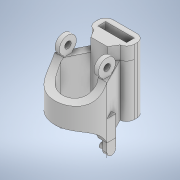
# Autodesk Inventor part: 손가락_중간
Saved by Autodesk Inventor 2022 (Build 260153000, 153)
## iProperties
Created: 2023-11-18
Part Number: 손가락_중간
Material: 일반
Document SubType Name: Modeling
Designer: USER
Density: 1 g/cm^3
Appearance: 기본값
Author: USER
Autodesk Inventor part; units mm, degrees
ref_plane "YZ Plane" through (0, 0, 0) normal (1, 0, 0) x (0, 1, 0)
ref_plane "XZ Plane" through (0, 0, 0) normal (0, 1, 0) x (-1, 0, 0)
sketch "스케치1" plane through (0, 0, 0) normal (0, 1, 0) x (-1, 0, 0)
  line L0 (0, 0) -> (0, -20)
  line L1 (0, -10) -> (-10, -10)
  line L2 (0, -20) -> (-5, -20)
  line L3 (-5, -20) -> (-10, -10)
  arc A0 (0, 0) -> (-10, -10) centre (0, -10) ccw
  line L4 (0, -20) -> (5, -20)
  line L5 (5, -20) -> (10, -10)
  arc A1 (10, -10) -> (0, 0) centre (0, -10) ccw
  dimension "d0" = 20
  dimension "d1" = 10
  dimension "d2" = 5
  constraints: 12 end point, 4 point on circle, 2 centre point, 2 horizontal, 2 symmetric about line, 1 coincident, 1 midpoint, 1 point on line, 1 vertical, 1 other
  measures "d0" distance of L0.start L0.end
  measures "d1" distance of L1.end L1.start
  measures "d2" distance of L0.end L2.end
extrude "돌출1" add sketch "스케치1" along normal blind 20
sketch "스케치2" plane through (0, 0, 0) normal (1, 0, 0) x (0, 1, 0)
  line L0 (0, 0) -> (20, 0) projected
  line L1 (20.0022, 0) -> (14.0022, 0)
  line L2 (25.6628, 0) -> (14.0022, 0)
  line L3 (10.0065, 0) -> (10.0065, 12.925)
  spline S0 degree 2 poles (14.0022, 0) (13.9613, -9.8069) (25.6628, -11.6913) knots 0 0 0 1 1 1
  line L4 (25.6628, -11.6913) -> (25.6628, 0)
  line L5 (0, -10) -> (20, -10) projected
  line L6 (0, -10) -> (28.6414, -10)
  line L7 (0, -10) -> (-10.0964, -10)
  line L8 (-5.6498, 0) -> (6.0108, 0)
  spline S1 degree 2 poles (6.0108, 0) (6.0517, -9.8069) (-5.6498, -11.6913) knots 0 0 0 1 1 1
  line L9 (-5.6498, -11.6913) -> (-5.6498, 0)
  point P0 (16.5578, -7.4686)
  point P1 (3.4551, -7.4686)
  point P2 (6.0108, 0)
  dimension "d5" = 6
  constraints: 16 end point, 4 symmetric about line, 3 point on line, 2 horizontal, 1 perpendicular, 1 vertical, 7 other
  measures "d5" distance of L1.start L1.end
shell "쉘1" thickness 3 removed faces 2 at (1.8644, 20, -8.0053) at (1.8644, 0, -8.0053)
extrude "돌출3" cut sketch "스케치2" along normal mid plane 30 contours L0 L1 L2 L4 L6 S0 | L6 L4 S0
sketch "스케치8" plane through (0, 20, 0) normal (0, 1, 0) x (1, 0, 0)
  arc A0 (-10, 10) -> (10, 10) centre (0, 10) ccw projected
  line L0 (-6.6459, 10) -> (-3.1459, 17) projected
  line L1 (-10, 10) -> (-6.6459, 10)
  line L2 (-8.3229, 10) -> (-8.3229, 13.3541)
  line L3 (-5, 20) -> (-10, 10) projected
  line L4 (-8.3229, 13.3541) -> (-6.6459, 13.3541)
  line L5 (-6.6459, 13.3541) -> (-6.6459, 10)
  line L6 (5, 20) -> (-5, 20) projected
  line L7 (0, 20) -> (0, 17)
  line L8 (-3.1459, 17) -> (3.1459, 17) projected
  line L9 (-8.3229, 10) -> (-6.6459, 10)
  line L10 (10, 10) -> (6.6459, 10)
  line L11 (8.3229, 10) -> (8.3229, 13.3541)
  line L12 (8.3229, 13.3541) -> (6.6459, 13.3541)
  line L13 (6.6459, 13.3541) -> (6.6459, 10)
  point P0 (0, 0)
  constraints: 20 end point, 4 symmetric about line, 3 horizontal, 3 midpoint, 1 perpendicular, 1 point on line, 1 vertical
extrude "돌출7" cut sketch "스케치2" along normal mid plane 30 contours L0 S1 L5 L7 L9 L8 | S1 L9 L7 L5
sketch "스케치9" plane through (0, 0, 0) normal (0, -1, 0) x (1, 0, 0)
  line L0 (9.9968, -10.0064) -> (5, -20) projected
  line L1 (6.6427, -10.0064) -> (3.1459, -17) projected
  line L2 (9.9968, -10.0064) -> (6.6427, -10.0064)
  line L3 (8.3198, -10.0064) -> (8.3198, -13.3605)
  line L4 (5, -20) -> (-5, -20) projected
  line L5 (0, -20) -> (0, -17)
  line L6 (-3.1459, -17) -> (3.1459, -17) projected
  line L7 (10, -10) -> (5, -20) projected
  line L8 (10, -10) -> (10, -13.3605)
  line L9 (10, -13.3605) -> (8.3198, -13.3605)
  line L10 (-9.9968, -10.0064) -> (-6.6427, -10.0064)
  line L11 (-5, -20) -> (-9.9968, -10.0064) projected
  line L12 (-9.9968, -10.0064) -> (-9.9968, -13.3605)
  line L13 (-9.9968, -13.3605) -> (-8.3198, -13.3605)
  line L14 (-8.3198, -13.3605) -> (-8.3198, -10.0064)
  point P0 (0, 0)
  constraints: 18 end point, 4 midpoint, 3 perpendicular, 3 symmetric about line, 2 vertical, 1 horizontal, 1 point on line
extrude "돌출8" add sketch "스케치8" along normal blind 5 contours L1 L2 L4 L5 | L10 L13 L12 L11
extrude "돌출9" add sketch "스케치9" along normal blind 5 contours L7 L8 L9 L0 | L0 L3 L2 | L10 L14 L11 | L11 L13 L12
sketch "스케치10" plane through (8.3229, 20, -10) normal (1, 0, 0) x (0, 0, -1)
  line L0 (10, 0) -> (3.3541, 0) projected
  line L1 (0, 5) -> (3.3541, 5)
  line L2 (3.3541, 5) -> (3.3541, 0)
  line L3 (3.3541, 0) -> (0, 0)
  line L4 (0, 0) -> (0, 5)
  circle A0 centre (1.6771, 3.3229) radius 3.25
  line L5 (3.3541, 0) -> (3.3541, 5) projected
  circle A1 centre (1.6771, 3.3229) radius 1.25
  point P0 (-10, -20)
  point P1 (0, 0.5391)
  point P2 (1.6771, 5)
  point P3 (3.3541, 0.5391)
  dimension "d28" = 6.5
  dimension "d29" = 2.5
  constraints: 8 end point, 2 centre point, 2 parallel, 1 coincident, 1 horizontal, 1 perpendicular
  measures "d28" diameter of A0
  measures "d29" diameter of A1
sketch "스케치11" plane through (0, 0, 0) normal (0, 1, 0) x (1, 0, 0)
  line L0 (-9.9968, 13.3605) -> (-8.3198, 13.3605) projected
  line L1 (-9.9968, 13.3605) -> (-8.3198, 13.3605)
  line L2 (-8.3198, 13.3605) -> (-9.9968, 10.0064) projected
  line L3 (-8.3198, 13.3605) -> (-9.9968, 10.0064)
  line L4 (-9.9968, 10.0064) -> (-9.9968, 13.3605) projected
  line L5 (-9.9968, 10.0064) -> (-9.9968, 13.3605)
  line L6 (8.3198, 13.3605) -> (10, 13.3605) projected
  line L7 (8.3198, 13.3605) -> (10, 13.3605)
  line L8 (9.9968, 10.0064) -> (8.3198, 13.3605) projected
  line L9 (10, 13.3605) -> (9.9968, 10.0064)
  line L10 (9.9968, 10.0064) -> (8.3198, 13.3605)
  point P0 (0, 0)
  constraints: 12 end point, 5 collinear
extrude "돌출10" add sketch "스케치11" along normal blind 8
sketch "스케치12" plane through (8.3198, 0, -13.3605) normal (-1, 0, 0) x (0, 0, 1)
  line L0 (0, 0) -> (3.3541, 0) projected
  line L1 (0, 0) -> (0, -5) projected
  line L2 (3.3541, 0) -> (0, 0)
  line L3 (0, 0) -> (0, -5)
  line L4 (0, -5) -> (3.3541, -5)
  line L5 (3.3541, -5) -> (3.3541, 0)
  circle A0 centre (1.6771, -3.3229) radius 1.6771
  line L6 (3.3541, 0) -> (3.3541, -5) projected
  line L7 (3.3541, -5) -> (0, -5) projected
  circle A1 centre (1.6771, -3.3229) radius 1
  point P0 (13.3605, 0)
  point P1 (3.3541, -3.3229)
  point P2 (1.6771, -5)
  point P3 (0, -3.3229)
  dimension "d32" = 2
  constraints: 8 end point, 2 centre point, 2 parallel, 2 tangent, 1 coincident, 1 horizontal, 1 perpendicular
  measures "d32" diameter of A1
extrude "돌출11" cut sketch "스케치12" along normal mid plane 100 contours A0 L4 L1 | L5 L4 A0
extrude "돌출12" add sketch "스케치12" along normal blind 2 contours A1
sketch "스케치13" plane through (-8.3198, 0, -10.0064) normal (1, 0, 0) x (0, 0, -1)
  arc A0 (0, -3.3229) -> (3.3541, -3.3229) centre (1.6771, -3.3229) ccw projected
  line L0 (3.3541, 0) -> (3.3541, -3.3229) projected
  line L1 (0, 0) -> (3.3541, 0) projected
  line L2 (0, 0) -> (0, -3.3229) projected
  line L3 (3.3541, -5) -> (0, -5) projected
  line L4 (0, 0) -> (0, -5) projected
  line L5 (3.3541, 0) -> (3.3541, -3.3229) projected
  line L6 (3.3541, 0) -> (3.3541, -5) projected
  arc A1 (0, -3.3229) -> (3.3541, -3.3229) centre (1.6771, -3.3229) ccw projected
  circle A2 centre (1.6771, -3.3229) radius 1.6771 projected
  circle A3 centre (1.6771, -3.3229) radius 1 projected
  point P0 (-10.0064, 0)
extrude "돌출13" add sketch "스케치13" along normal blind 2 contours A3
sketch "스케치14" plane through (-6.6459, 20, -10) normal (1, 0, 0) x (0, 0, -1)
  circle A0 centre (1.6771, 3.3229) radius 1.25 projected
  circle A1 centre (1.6771, 3.3229) radius 3.25
  point P0 (-10, -20)
  dimension "d56" = 6.5
  constraints: 1 centre point, 1 coincident
  measures "d56" diameter of A1
sketch "스케치15" plane through (0, 20, 0) normal (0, 1, 0) x (1, 0, 0)
  line L0 (5, 20) -> (-5, 20) projected
  line L1 (-5, 20) -> (5, 20)
  line L2 (-3.1459, 17) -> (3.1459, 17) projected
  line L3 (5, 20) -> (3.1459, 17)
  line L4 (3.1459, 17) -> (-3.1459, 17)
  line L5 (-5, 20) -> (-8.3229, 13.3541) projected
  line L6 (-3.1459, 17) -> (-5, 20)
  point P0 (0, 0)
  constraints: 8 end point, 2 collinear
extrude "돌출15" add sketch "스케치15" along normal blind 5
ref_plane "작업 평면1" through (0, 25, 0) normal (0, 1, 0) x (1, 0, 0)
sketch "스케치16" plane through (0, 25, 0) normal (0, 1, 0) x (1, 0, 0)
  line L0 (-5, 20) -> (-3.1459, 17) projected
  line L1 (3.1459, 17) -> (5, 20) projected
  line L2 (-5, 20) -> (5, 20)
  line L3 (-7.5, 27) -> (7.5, 27)
  line L4 (7.5, 27) -> (7.5, 20)
  line L5 (7.5, 20) -> (-7.5, 20)
  line L6 (-7.5, 20) -> (-7.5, 27)
  line L7 (5.5, 25) -> (-5.5, 25)
  line L8 (-5.5, 25) -> (-5.5, 22)
  line L9 (-5.5, 22) -> (5.5, 22)
  line L10 (5.5, 22) -> (5.5, 25)
  point P0 (0, 0)
  dimension "d44" = 7
  dimension "d45" = 15
  dimension "d46" = 2.5
  dimension "d47" = 0
  dimension "d48" = 2
  constraints: 18 end point, 4 parallel, 2 horizontal, 2 perpendicular, 3 other
  measures "d44" distance of L3.end L4.end
  measures "d45" distance of L4.end L5.end
  measures "d46" distance of L0.start L5.end
  measures "d47" distance between parallel lines of L2 L5
  measures "d48" distance between parallel lines of L3 L7
extrude "돌출16" add sketch "스케치16" against normal blind 25
fillet "모깎기1" radius 3 4 edges at (7.5, 12.5, -27) (-7.5, 12.5, -27) (-7.5, 12.5, -20) (7.5, 12.5, -20)
extrude "돌출17" add sketch "스케치10" against normal blind 1.677 contours L4 A0 L2 L1 picked at (1.7841, 5.519)
extrude "돌출18" cut sketch "스케치10" against normal blind 1.677 contours A1
extrude "돌출19" add sketch "스케치14" against normal blind 1.677
extrude "돌출20" cut sketch "스케치14" against normal blind 1.677 contours A0
extrude "돌출21" cut sketch "스케치14" along normal mid plane 50 contours A0
